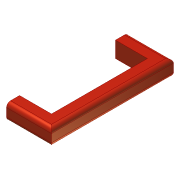
# Autodesk Inventor part: BumperRepresentation
Saved by Autodesk Inventor 2012 (Build 160160000, 160)
## iProperties
Created: 2013-01-07
Part Number: BumperRepresentation
Material: Default
Document SubType Name: Modeling
Designer: JesseK
Density: 2.71263 g/cm^3
Mass: 3401.94 g
Surface Area: 3813.2 cm^2
Volume: 7849.31 cm^3
Author: JesseK
Autodesk Inventor part; units mm, degrees
ref_plane "YZ Plane" through (0, 0, 0) normal (1, 0, 0) x (0, 1, 0)
ref_plane "XZ Plane" through (0, 0, 0) normal (0, 1, 0) x (-1, 0, 0)
ref_plane "XY Plane" through (0, 0, 0) normal (0, 0, 1) x (1, 0, 0)
sketch "Sketch2" plane through (0, 0, 0) normal (0, 1, 0) x (-1, 0, 0)
  line L0 (0, 0) -> (-285.75, 0)
  line L1 (-285.75, 0) -> (-285.75, 774.7)
  line L2 (-285.75, 774.7) -> (0, 774.7)
  line L3 (0, 774.7) -> (0, 692.15)
  line L4 (0, 692.15) -> (-203.2, 692.15)
  line L5 (-203.2, 692.15) -> (-203.2, 82.55)
  line L6 (-203.2, 82.55) -> (0, 82.55)
  line L7 (0, 82.55) -> (0, 0)
  dimension "d0" = 82.55
  dimension "d1" = 203.2
  dimension "d2" = 82.55
  dimension "d4" = 609.6
  constraints: 16 end point, 4 horizontal, 4 vertical, 2 collinear
  measures "d0" distance of L6.end L0.start
  measures "d1" distance of L3.end L4.end
  measures "d2" distance between parallel lines of L5 L1
  measures "d4" distance between parallel lines of L6 L4
extrude "Extrusion1" add sketch "Sketch2" along normal blind 101.6
fillet "Fillet1" radius 25.4 6 edges at (285.75, 101.6, 387.35) (285.75, 0, 387.35) (142.875, 101.6, 0) (142.875, 101.6, 774.7) (142.875, 0, 774.7) (142.875, 0, 0)
body "Solid1"
